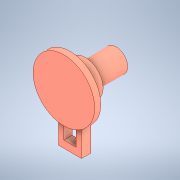
# Autodesk Inventor part: innerGear1
Saved by Autodesk Inventor 2020.1 (Build 241239000, 239)
## iProperties
Created: 2020-01-18
Part Number: innerGear1
Material: Generic
Document SubType Name: Modeling
Designer: Ali
Density: 1 g/cm^3
Appearance: Default
Author: Ali
Autodesk Inventor part; units mm, degrees
ref_plane "YZ Plane" through (0, 0, 0) normal (1, 0, 0) x (0, 1, 0)
ref_plane "XZ Plane" through (0, 0, 0) normal (0, 1, 0) x (-1, 0, 0)
ref_plane "XY Plane" through (0, 0, 0) normal (0, 0, 1) x (1, 0, 0)
sketch "Sketch1" plane through (0, 0, 0) normal (0, 0, 1) x (1, 0, 0)
  circle A0 centre (0, 0) radius 10
  dimension "d0" = 20
  constraints: 1 centre point, 1 coincident
  measures "d0" diameter of A0
extrude "Extrusion1" add sketch "Sketch1" along normal blind 2
sketch "Sketch2" plane through (0, 0, 2) normal (0, 0, 1) x (1, 0, 0)
  circle A0 centre (0, 0) radius 3.75
  dimension "d3" = 7.5
  constraints: 1 centre point, 1 coincident
  measures "d3" diameter of A0
extrude "Extrusion2" add sketch "Sketch2" along normal blind 15
ref_plane "Work Plane2" through (0, 0, 7) normal (0, 0, 1) x (1, 0, 0)
sketch "Sketch7" plane through (0, 0, 7) normal (0, 0, 1) x (1, 0, 0)
  circle A0 centre (0, 0) radius 3.75 projected
  circle A1 centre (0, 0) radius 5.75
  dimension "d27" = 2
  constraints: 1 centre point
  measures "d27" radial gap between concentric circles of A1 A0
extrude "Extrusion7" add sketch "Sketch7" against normal blind 2
sketch "Sketch8" plane through (0, 0, 5) normal (0, 0, -1) x (-1, 0, 0)
  circle A0 centre (0, 0) radius 5.75 projected
  circle A1 centre (0, 0) radius 3.75 projected
  circle A2 centre (0, 0) radius 5.75 construction
  line L0 (5.75, 0) -> (-5.75, 0) construction
  line L1 (-3.75, 0) -> (3.75, 0)
  line L2 (3.75, 0) -> (3.75, -18.3333)
  line L3 (3.75, -18.3333) -> (-3.75, -18.3333)
  line L4 (-3.75, -18.3333) -> (-3.75, 0)
  dimension "d31" = 18.3333
  constraints: 10 end point, 2 horizontal, 2 parallel, 2 point on circle, 1 perpendicular, 1 point on line, 2 other
  measures "d31" distance of L1.end L2.end
extrude "Extrusion8" add sketch "Sketch8" along normal blind 3 contours L4 A1 L2 A0 | A0 L2 L3 L4 picked at (2.8343, -4.1874)
sketch "Sketch9" plane through (0, 0, 2) normal (0, 0, -1) x (-1, 0, 0)
  arc A0 (-3.75, -4.3589) -> (3.75, -4.3589) centre (0, 0) ccw projected
  line L0 (3.75, -18.3333) -> (3.75, -4.3589) projected
  line L1 (-3.75, -18.3333) -> (3.75, -18.3333) projected
  line L2 (-3.75, -4.3589) -> (-3.75, -18.3333) projected
  line L3 (-2, -8) -> (2, -8)
  line L4 (2, -8) -> (2, -16)
  line L5 (2, -16) -> (-2, -16)
  line L6 (-2, -16) -> (-2, -8)
  dimension "d34" = 2
  dimension "d35" = 4
  dimension "d36" = 8
  dimension "d37" = 8
  constraints: 8 end point, 2 parallel, 1 horizontal, 1 perpendicular
  measures "d34" distance from line of point (0, 0) L6
  measures "d35" distance of L4.end L5.end
  measures "d36" distance between parallel lines of L5 L3
  measures "d37" distance from line of point (0, 0) L3
extrude "Extrusion9" cut sketch "Sketch9" against normal up to surface (3 mm away) draft 2 contours L3 L4 L5 L6
fillet "Fillet2" radius 0.25 4 edges at (0, -16.1048, 5) (2.1048, -12, 5) (-2.1048, -12, 5) (0, -7.8952, 5)
equation "\"d1\" = IG_gearThickness"
equation "\"d3\" = IG_shaftDiameter"
equation "\"d4\" = IG_shaftLength"
equation "\"Wheel_Related_W_\" = 0"
equation "\"W_innerDepth\" = 4"
equation "\"W_wallThickness\" = 2"
equation "\"W_holesClearance\" = 0.3"
equation "\"W_outerGearHoleDiameter\" = 5.3"
equation "\"W_innerGearHoleDiameter\" = 10.1"
equation "\"TempSpotReserved7\" = 0"
equation "\"TempSpotReserved8\" = 0"
equation "\"TempSpotReserved9\" = 0"
equation "\"TempSpotReserved10\" = 0"
equation "\"TempSpotReserved11\" = 0"
equation "\"TempSpotReserved12\" = 0"
equation "\"TempSpotReserved13\" = 0"
equation "\"TempSpotReserved14\" = 0"
equation "\"TempSpotReserved15\" = 0"
equation "\"TempSpotReserved16\" = 0"
equation "\"TempSpotReserved17\" = 0"
equation "\"TempSpotReserved18\" = 0"
equation "\"TempSpotReserved19\" = 0"
equation "\"TempSpotReserved20\" = 0"
equation "\"Inner_Gear_Related_IG_\" = 0"
equation "\"IG_shaftDiameter\" = 7.5"
equation "\"IG_shaftLength\" = 15"
equation "\"IG_gearThickness\" = 2"
equation "\"TempSpotReserved25\" = 0"
equation "\"TempSpotReserved26\" = 0"
equation "\"TempSpotReserved27\" = 0"
equation "\"TempSpotReserved28\" = 0"
equation "\"TempSpotReserved29\" = 0"
equation "\"TempSpotReserved30\" = 0"
equation "\"TempSpotReserved31\" = 0"
equation "\"TempSpotReserved32\" = 0"
equation "\"TempSpotReserved33\" = 0"
equation "\"TempSpotReserved34\" = 0"
equation "\"TempSpotReserved35\" = 0"
equation "\"TempSpotReserved36\" = 0"
equation "\"TempSpotReserved37\" = 0"
equation "\"TempSpotReserved38\" = 0"
equation "\"TempSpotReserved39\" = 0"
equation "\"TempSpotReserved40\" = 0"
equation "\"Outer_Gear_Related_OG_\" = 0"
equation "\"OG_distanceFromCenter\" = 23.33333"
equation "\"OG_shaftDiameter\" = 5"
equation "\"OG_gearDiameter\" = 26.66667"
equation "\"OG_shaftLength\" = 7"
equation "\"OG_gearThickness\" = 2"
equation "\"TempSpotReserved47\" = 0"
equation "\"TempSpotReserved48\" = 0"
equation "\"TempSpotReserved49\" = 0"
equation "\"TempSpotReserved50\" = 0"
equation "\"TempSpotReserved51\" = 0"
equation "\"TempSpotReserved52\" = 0"
equation "\"TempSpotReserved53\" = 0"
equation "\"TempSpotReserved54\" = 0"
equation "\"TempSpotReserved55\" = 0"
equation "\"TempSpotReserved56\" = 0"
equation "\"TempSpotReserved57\" = 0"
equation "\"TempSpotReserved58\" = 0"
equation "\"TempSpotReserved59\" = 0"
equation "\"TempSpotReserved60\" = 0"
equation "\"Leg_Extensions_Related_LE_\" = 0"
equation "\"LE_baseDiameter\" = 5"
equation "\"LE_maxLength\" = 24.6522"
equation "\"LE_thickness\" = 2.5"
equation "\"IG_ratioToOuterGear\" = 0.75"
equation "\"B_bearingThickness\" = 1"
equation "\"TempSpotReserved43\" = 0"
equation "\"TempSpotReserved45\" = 0"
equation "\"Thisisatest\" = 25.4"
equation "\"TempSpotReserved46\" = 0"
equation "\"TempSpotReserved44\" = 0"
equation "\"LE_offsetAboveOuterGear\" = 0"
equation "\"Bearing_Related_B_\" = 0"
equation "\"TempSpotReserved42\" = 0"
equation "\"OG_skirtOffset\" = 1"
equation "\"OG_skirtThickness\" = 1"
equation "\"IG_skirtThickness\" = 2"
equation "\"IG_extentionLength\" = 18.33333"
equation "\"IG_extentionThickness\" = 3"
equation "\"IG_slitWidth\" = 4"
equation "\"IG_slitlength\" = 8"
equation "\"IG_slitDistanceFromCenterHole\" = 8"
equation "\"IG_slitClearance\" = 0.2"
equation "\"Reserved_10\" = 0"
equation "\"Reserved_9\" = 0"
equation "\"Reserved_11\" = 0"
equation "\"Reserved_12\" = 0"
equation "\"Reserved_8\" = 0"
equation "\"Reserved_7\" = 0"
equation "\"Reserved_26\" = 0"
equation "\"Reserved_20\" = 0"
equation "\"Reserved_22\" = 0"
equation "\"Reserved_23\" = 0"
equation "\"Reserved_25\" = 0"
equation "\"Reserved_24\" = 0"
equation "\"Reserved_21\" = 0"
equation "\"Reserved_19\" = 0"
equation "\"Reserved_27\" = 0"
equation "\"Reserved_14\" = 0"
equation "\"Reserved_15\" = 0"
equation "\"Reserved_16\" = 0"
equation "\"Reserved_13\" = 0"
equation "\"Reserved_17\" = 0"
equation "\"Reserved_18\" = 0"
equation "\"Bearing_Related_BR_\" = 0"
equation "\"BR_bearingThickness\" = 1"
equation "\"Block_Related_BL_\" = 0"
equation "\"BL_width\" = 3.8"
equation "\"BL_length\" = 7.8"
equation "\"W_filletRadius\" = 0.25"
equation "\"W_extrutsionTaperAngle\" = 2deg"
equation "\"OG_protrudeDistance\" = 3"
body "Solid1"
